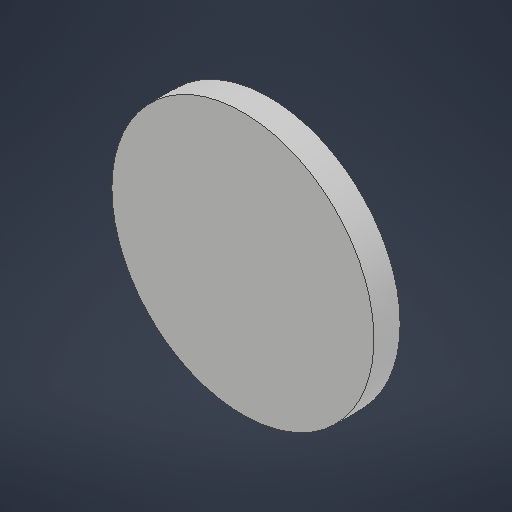
# Autodesk Inventor part: Tag
Saved by Autodesk Inventor 2026.1 (Build 301233020, 233B)
## iProperties
Created: 2026-04-07
Part Number: Tag
Material: Generic
Document SubType Name: Modeling
Designer: Bahaa
Mass: 2.03922 g
Surface Area: 17.2217 cm^2
Volume: 2.03922 cm^3
Density: 1 g/cm^3
Appearance: Default
Mass: 1.90866 g
Surface Area: 18.2937 cm^2
Volume: 1.90866 cm^3
Author: Bahaa
Autodesk Inventor part; units mm, degrees
ref_plane "YZ Plane" through (0, 0, 0) normal (1, 0, 0) x (0, 1, 0)
ref_plane "XZ Plane" through (0, 0, 0) normal (0, 1, 0) x (-1, 0, 0)
ref_plane "XY Plane" through (0, 0, 0) normal (0, 0, 1) x (1, 0, 0)
sketch "Sketch1" plane through (0, 0, 0) normal (0, 1, 0) x (-1, 0, 0)
  circle A0 centre (0, 0) radius 15
  dimension "d0" = 30
  constraints: 1 centre point, 1 coincident
  measures "d0" diameter of A0
extrude "Extrusion1" add sketch "Sketch1" against normal blind 2.8
sketch "Sketch2" plane through (0, 0, 0) normal (0, 1, 0) x (1, 0, 0)
  line L0 (7.5, -7.5) -> (-7.5, -7.5)
  line L1 (-7.5, -7.5) -> (-7.5, 7.5)
  line L2 (-7.5, 7.5) -> (7.5, 7.5)
  line L3 (7.5, 7.5) -> (7.5, -7.5)
  line L4 (7.5, -7.5) -> (-7.5, 7.5) construction
  line L5 (-7.5, -7.5) -> (7.5, 7.5) construction
  circle A0 centre (0, 0) radius 12
  circle A1 centre (0, 0) radius 15 projected
  spline S0 degree 2 poles (6.3976, -3.7402) (6.2555, -3.773) (5.8727, -3.773) (5.7524, -3.773) knots 0 0 0 1 2 2 2
  spline S1 degree 2 poles (5.7524, -3.773) (4.615, -3.773) (2.7559, -2.8106) (1.1592, -1.367) (0.4593, -0.6452) knots 0 0 0 1 2 3 3 3
  spline S2 degree 2 poles (0.4593, -0.6452) (-0.0766, -0.0766) (-1.1264, 0.9186) (-2.1872, 1.5201) (-2.7668, 1.5201) knots 0 0 0 1 2 3 3 3
  spline S3 degree 2 poles (-2.7668, 1.5201) (-3.7292, 1.5201) (-4.626, 0.3937) (-4.626, -0.4156) knots 0 0 0 1 2 2 2
  spline S4 degree 2 poles (-4.626, -0.4156) (-4.626, -0.9952) (-4.2542, -1.9685) (-3.7073, -2.745) (-3.4339, -3.0293) knots 0 0 0 1 2 3 3 3
  line L6 (-3.4339, -3.0293) -> (-4.8228, -4.0026)
  spline S5 degree 2 poles (-4.8228, -4.0026) (-5.2056, -3.6636) (-5.9493, -2.5481) (-6.3976, -1.1045) (-6.3976, -0.3062) knots 0 0 0 1 2 3 3 3
  spline S6 degree 2 poles (-6.3976, -0.3062) (-6.3976, 0.8858) (-5.5993, 2.6137) (-4.0354, 3.5324) (-2.8762, 3.5324) knots 0 0 0 1 2 3 3 3
  spline S7 degree 2 poles (-2.8762, 3.5324) (-2.0341, 3.5324) (-0.4374, 2.7122) (1.0389, 1.3889) (1.7607, 0.6671) knots 0 0 0 1 2 3 3 3
  spline S8 degree 2 poles (1.7607, 0.6671) (2.0341, 0.3828) (2.8106, -0.3828) (3.6417, -1.0608) (4.4073, -1.5201) (4.7244, -1.5201) knots 0 0 0 1 2 3 4 4 4
  line L7 (4.7244, -1.5201) -> (4.7244, 4.0792)
  line L8 (4.7244, 4.0792) -> (6.3976, 4.0792)
  line L9 (6.3976, 4.0792) -> (6.3976, -3.7402)
  dimension "d3" = 15
  dimension "d4" = 15
  dimension "d13" = 3
  constraints: 12 end point, 2 coincident, 2 midpoint, 2 parallel, 1 centre point, 1 horizontal, 1 perpendicular, 1 other
  measures "d3" distance of L1.end L2.end
  measures "d4" distance of L0.end L1.end
  measures "d13" radial gap between concentric circles of A1 A0
extrude "Extrusion2" add sketch "Sketch2" along normal blind 0.2 contours A1 | S0 S1 S2 S3 S4 L6 S5 S6 S7 S8 L7 L8 L9
body "Solid1"
